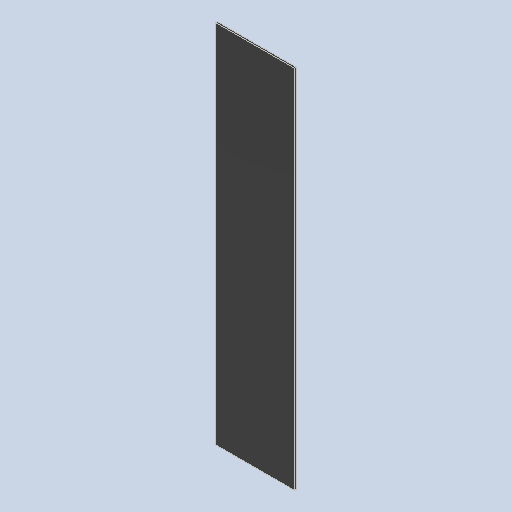
# Autodesk Inventor part: BodyCover
Saved by Autodesk Inventor 2023 (Build 270158000, 158)
## iProperties
Created: 2022-03-03
Part Number: BodyCover
Material: Generic
Document SubType Name: Modeling
Designer: Jochen
Density: 1 g/cm^3
Appearance: Sky Blue Dark
Author: Jochen
Autodesk Inventor part; units mm, degrees
ref_plane "YZ Plane" through (0, 0, 0) normal (1, 0, 0) x (0, 1, 0)
ref_plane "XZ Plane" through (0, 0, 0) normal (0, 1, 0) x (-1, 0, 0)
ref_plane "XY Plane" through (0, 0, 0) normal (0, 0, 1) x (1, 0, 0)
sketch "Sketch1" plane through (0, 0, 0) normal (0, 0, 1) x (1, 0, 0)
  line L0 (0, -288.4) -> (0, 288.4) construction
  line L1 (-62.3, 0) -> (62.3, 0) construction
  line L2 (44.5, -206) -> (-44.5, -206)
  line L3 (-44.5, -206) -> (-44.5, 206)
  line L4 (-44.5, 206) -> (44.5, 206)
  line L5 (44.5, 206) -> (44.5, -206)
  line L6 (44.5, -206) -> (-44.5, 206) construction
  line L7 (-44.5, -206) -> (44.5, 206) construction
  point P0 (0, 0)
  dimension "d0" = 89
  dimension "d1" = 412
  constraints: 12 end point, 2 midpoint, 2 parallel, 1 horizontal, 1 perpendicular
  measures "d0" distance of L3.end L4.end
  measures "d1" distance of L2.end L3.end
extrude "Extrusion1" add sketch "Sketch1" along normal blind 2
body "Solid1"
